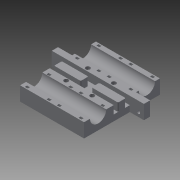
# Autodesk Inventor part: x-carriage
Saved by Autodesk Inventor 2015 SP2 (Build 190223200, 223)
## iProperties
Created: 2016-02-13
Part Number: x-carriage
Material: Generic
Document SubType Name: Modeling
Designer: marc
Density: 1 g/cm^3
Appearance: Default
Author: marc
Autodesk Inventor part; units mm, degrees
ref_plane "YZ Plane" through (0, 0, 0) normal (1, 0, 0) x (0, 1, 0)
ref_plane "XZ Plane" through (0, 0, 0) normal (0, 1, 0) x (-1, 0, 0)
ref_plane "XY Plane" through (0, 0, 0) normal (0, 0, 1) x (1, 0, 0)
sketch "Sketch1" plane through (0, 0, 0) normal (0, 0, 1) x (1, 0, 0)
  line L0 (-42.5, -35) -> (42.5, -35)
  line L1 (42.5, -35) -> (42.5, 35)
  line L2 (42.5, 35) -> (-42.5, 35)
  line L3 (-42.5, 35) -> (-42.5, -35)
  line L4 (-42.5, -35) -> (42.5, 35) construction
  line L5 (42.5, -35) -> (-42.5, 35) construction
  point P0 (0, 0)
  dimension "d0" = 85
  dimension "d1" = 70
  constraints: 12 end point, 2 midpoint, 2 parallel, 1 horizontal, 1 perpendicular
  measures "d0" distance of L1.end L2.end
  measures "d1" distance between parallel lines of L0 L2
extrude "Extrusion1" add sketch "Sketch1" along normal blind 13
sketch "Sketch2" plane through (0, 0, 13) normal (0, 0, 1) x (1, 0, 0)
  line L0 (-42.5, 35) -> (-29.5, 35)
  line L1 (-29.5, 35) -> (-29.5, 13)
  line L2 (-29.5, 13) -> (-42.5, 13)
  line L3 (-42.5, 13) -> (-42.5, 35)
  line L4 (-42.5, -35) -> (-29.5, -35)
  line L5 (-29.5, -35) -> (-29.5, 7.25)
  line L6 (-29.5, 7.25) -> (-42.5, 7.25)
  line L7 (-42.5, 7.25) -> (-42.5, -35)
  line L8 (42.5, 35) -> (-42.5, 35) construction
  line L9 (0, 35) -> (0, -35) construction
  line L10 (-42.5, -35) -> (42.5, -35) construction
  line L11 (42.5, 35) -> (29.5, 35)
  line L12 (29.5, 35) -> (29.5, 13)
  line L13 (29.5, 13) -> (42.5, 13)
  line L14 (42.5, 13) -> (42.5, 35)
  line L15 (42.5, -35) -> (29.5, -35)
  line L16 (29.5, -35) -> (29.5, 7.25)
  line L17 (29.5, 7.25) -> (42.5, 7.25)
  line L18 (42.5, 7.25) -> (42.5, -35)
  point P0 (0, 0)
  dimension "d4" = 13
  dimension "d5" = 5.75
  dimension "d6" = 22
  constraints: 34 end point, 6 symmetric about line, 4 parallel, 2 horizontal, 2 midpoint, 2 perpendicular, 2 point on line
  measures "d4" distance of L1.end L2.end
  measures "d5" distance between parallel lines of L6 L2
  measures "d6" distance of L0.end L1.end
extrude "Extrusion2" cut sketch "Sketch2" against normal through all
sketch "Sketch3" plane through (29.5, 13, 13) normal (1, 0, 0) x (0, 0, -1)
  circle A0 centre (0, 10) radius 7.5
  circle A1 centre (0, -35) radius 7.5
  line L0 (0, 10) -> (0, -35) construction
  line L1 (0, -48) -> (0, -5.75) construction
  line L2 (0, 0) -> (0, 22) construction
  line L3 (0, 22) -> (13, 22) construction
  point P0 (13, -13)
  dimension "d9" = 15
  dimension "d10" = 15
  dimension "d11" = 45
  dimension "d12" = 12
  constraints: 2 centre point, 2 end point, 1 collinear, 1 point on line, 1 vertical
  measures "d9" diameter of A0
  measures "d10" diameter of A1
  measures "d11" distance of L0.end L0.start
  measures "d12" distance from line of L0.start L3
extrude "Extrusion3" cut sketch "Sketch3" against normal through all
sketch "Sketch4" plane through (0, 0, 13) normal (0, 0, 1) x (1, 0, 0)
  line L0 (-12, -10) -> (12, -10) construction
  line L1 (12, -10) -> (12, 10) construction
  line L2 (12, 10) -> (-12, 10) construction
  line L3 (-12, 10) -> (-12, -10) construction
  line L4 (-12, -10) -> (12, 10) construction
  line L5 (12, -10) -> (-12, 10) construction
  point P0 (0, 0)
  dimension "d15" = 24
  dimension "d16" = 20
  constraints: 12 end point, 4 coincident, 2 midpoint, 2 parallel, 1 horizontal, 1 perpendicular
  measures "d15" distance between parallel lines of L1 L3
  measures "d16" distance between parallel lines of L0 L2
hole "Hole1" at (-12, 10, 13) at (12, 10, 13) at (12, -10, 13) at (-12, -10, 13) direction (0, 0, -1) diameter 4 end through all
sketch "Sketch6" plane through (0, 0, 13) normal (0, 0, 1) x (1, 0, 0)
  line L0 (0, -28.0217) -> (0, 47.4955) construction
  line L1 (-24.75, 13) -> (-4.75, 13) construction
  line L2 (-4.75, 13) -> (-4.75, 33) construction
  line L3 (-4.75, 33) -> (-24.75, 33) construction
  line L4 (-24.75, 33) -> (-24.75, 13) construction
  line L5 (-24.75, 13) -> (-4.75, 33) construction
  line L6 (-4.75, 13) -> (-24.75, 33) construction
  line L7 (-26.1, 32) -> (-23.4, 32)
  line L8 (-23.4, 32) -> (-23.4, 34)
  line L9 (-23.4, 34) -> (-26.1, 34)
  line L10 (-26.1, 34) -> (-26.1, 32)
  line L11 (-26.1, 32) -> (-23.4, 34) construction
  line L12 (-23.4, 32) -> (-26.1, 34) construction
  line L13 (-6.1, 32) -> (-3.4, 32)
  line L14 (-3.4, 32) -> (-3.4, 34)
  line L15 (-3.4, 34) -> (-6.1, 34)
  line L16 (-6.1, 34) -> (-6.1, 32)
  line L17 (-6.1, 32) -> (-3.4, 34) construction
  line L18 (-3.4, 32) -> (-6.1, 34) construction
  line L19 (-26.1, 12) -> (-23.4, 12)
  line L20 (-23.4, 12) -> (-23.4, 14)
  line L21 (-23.4, 14) -> (-26.1, 14)
  line L22 (-26.1, 14) -> (-26.1, 12)
  line L23 (-26.1, 12) -> (-23.4, 14) construction
  line L24 (-23.4, 12) -> (-26.1, 14) construction
  line L25 (-6.1, 12) -> (-3.4, 12)
  line L26 (-3.4, 12) -> (-3.4, 14)
  line L27 (-3.4, 14) -> (-6.1, 14)
  line L28 (-6.1, 14) -> (-6.1, 12)
  line L29 (-6.1, 12) -> (-3.4, 14) construction
  line L30 (-3.4, 12) -> (-6.1, 14) construction
  line L31 (-24.75, -33) -> (-4.75, -33) construction
  line L32 (-4.75, -33) -> (-4.75, -13) construction
  line L33 (-4.75, -13) -> (-24.75, -13) construction
  line L34 (-24.75, -13) -> (-24.75, -33) construction
  line L35 (-24.75, -33) -> (-4.75, -13) construction
  line L36 (-4.75, -33) -> (-24.75, -13) construction
  line L37 (-6.1, -14) -> (-3.4, -14)
  line L38 (-3.4, -14) -> (-3.4, -12)
  line L39 (-3.4, -12) -> (-6.1, -12)
  line L40 (-6.1, -12) -> (-6.1, -14)
  line L41 (-6.1, -14) -> (-3.4, -12) construction
  line L42 (-3.4, -14) -> (-6.1, -12) construction
  line L43 (-26.1, -14) -> (-23.4, -14)
  line L44 (-23.4, -14) -> (-23.4, -12)
  line L45 (-23.4, -12) -> (-26.1, -12)
  line L46 (-26.1, -12) -> (-26.1, -14)
  line L47 (-26.1, -14) -> (-23.4, -12) construction
  line L48 (-23.4, -14) -> (-26.1, -12) construction
  line L49 (-26.1, -34) -> (-23.4, -34)
  line L50 (-23.4, -34) -> (-23.4, -32)
  line L51 (-23.4, -32) -> (-26.1, -32)
  line L52 (-26.1, -32) -> (-26.1, -34)
  line L53 (-26.1, -34) -> (-23.4, -32) construction
  line L54 (-23.4, -34) -> (-26.1, -32) construction
  line L55 (-6.1, -34) -> (-3.4, -34)
  line L56 (-3.4, -34) -> (-3.4, -32)
  line L57 (-3.4, -32) -> (-6.1, -32)
  line L58 (-6.1, -32) -> (-6.1, -34)
  line L59 (-6.1, -34) -> (-3.4, -32) construction
  line L60 (-3.4, -34) -> (-6.1, -32) construction
  line L61 (26.1, 32) -> (23.4, 32)
  line L62 (23.4, 32) -> (23.4, 34)
  line L63 (23.4, 34) -> (26.1, 34)
  line L64 (26.1, 34) -> (26.1, 32)
  line L65 (6.1, 32) -> (3.4, 32)
  line L66 (3.4, 32) -> (3.4, 34)
  line L67 (3.4, 34) -> (6.1, 34)
  line L68 (6.1, 34) -> (6.1, 32)
  line L69 (26.1, 12) -> (23.4, 12)
  line L70 (23.4, 12) -> (23.4, 14)
  line L71 (23.4, 14) -> (26.1, 14)
  line L72 (26.1, 14) -> (26.1, 12)
  line L73 (6.1, 12) -> (3.4, 12)
  line L74 (3.4, 12) -> (3.4, 14)
  line L75 (3.4, 14) -> (6.1, 14)
  line L76 (6.1, 14) -> (6.1, 12)
  line L77 (6.1, -14) -> (3.4, -14)
  line L78 (3.4, -14) -> (3.4, -12)
  line L79 (3.4, -12) -> (6.1, -12)
  line L80 (6.1, -12) -> (6.1, -14)
  line L81 (26.1, -14) -> (23.4, -14)
  line L82 (23.4, -14) -> (23.4, -12)
  line L83 (23.4, -12) -> (26.1, -12)
  line L84 (26.1, -12) -> (26.1, -14)
  line L85 (26.1, -34) -> (23.4, -34)
  line L86 (23.4, -34) -> (23.4, -32)
  line L87 (23.4, -32) -> (26.1, -32)
  line L88 (26.1, -32) -> (26.1, -34)
  line L89 (6.1, -34) -> (3.4, -34)
  line L90 (3.4, -34) -> (3.4, -32)
  line L91 (3.4, -32) -> (6.1, -32)
  line L92 (6.1, -32) -> (6.1, -34)
  point P0 (0, 0)
  point P1 (-14.75, 23)
  point P2 (-14.75, -23)
  dimension "d24" = 14.75
  dimension "d25" = 23
  dimension "d26" = 20
  dimension "d27" = 20
  dimension "d28" = 2.7
  dimension "d29" = 2
  dimension "d30" = 14.75
  dimension "d31" = 20
  dimension "d32" = 20
  dimension "d33" = 23
  dimension "d34" = 2.7
  dimension "d35" = 2
  constraints: 186 end point, 32 symmetric about line, 20 midpoint, 20 parallel, 10 horizontal, 10 perpendicular, 9 equal length, 7 point on line, 1 vertical
  measures "d24" distance from line of L0 point (-14.75, 23)
  measures "d25" vertical distance of point (0, 0) point (-14.75, 23)
  measures "d26" distance of L3.end L1.start
  measures "d27" distance between parallel lines of L2 L4
  measures "d28" distance of L8.end L9.end
  measures "d29" distance between parallel lines of L7 L9
  measures "d30" distance from line of L0 point (-14.75, -23)
  measures "d31" distance of L31.start L31.end
  measures "d32" distance between parallel lines of L31 L33
  measures "d33" vertical distance of point (0, 0) point (-14.75, -23)
  measures "d34" distance of L44.end L45.end
  measures "d35" distance between parallel lines of L43 L45
extrude "Extrusion4" cut sketch "Sketch6" against normal through all
sketch "Sketch7" plane through (0, 0, 13) normal (0, 0, 1) x (1, 0, 0)
  line L0 (-42.3851, 7.25) -> (42.4952, 7.25) construction
  line L1 (-42.5, 7.25) -> (-29.5, 7.25) projected
  line L2 (-42.3851, 0) -> (42.4952, 0) construction
  line L3 (-29.5, 7.25) -> (-29.5, -14.5) projected
  line L4 (-29.5, 3.5) -> (-5, 3.5)
  line L5 (-5, 3.5) -> (-5, -3.625)
  line L6 (-5, -3.625) -> (-29.5, -3.625)
  line L7 (-29.5, -3.625) -> (-29.5, -7.625)
  line L8 (-29.5, -7.625) -> (29.5, -7.625)
  line L9 (29.5, 7.25) -> (29.5, -35) projected
  line L10 (29.5, -7.625) -> (29.5, -3.625)
  line L11 (29.5, -3.625) -> (5, -3.625)
  line L12 (5, -3.625) -> (5, 3.5)
  line L13 (5, 3.5) -> (29.5, 3.5)
  line L14 (29.5, 3.5) -> (29.5, 7.25)
  line L15 (29.5, 7.25) -> (-29.5, 7.25)
  line L16 (-29.5, 7.25) -> (-29.5, 3.5)
  line L17 (0, 0) -> (0, 21.6097) construction
  dimension "d40" = 4
  dimension "d42" = 5
  dimension "d57" = 3.75
  constraints: 30 end point, 10 point on line, 4 collinear, 4 horizontal, 4 perpendicular, 1 midpoint, 1 vertical, 1 other
  measures "d40" distance between parallel lines of L8 L6
  measures "d42" distance from line of L17.start L5
  measures "d57" distance between parallel lines of L4 L0
extrude "Extrusion5" cut sketch "Sketch7" against normal blind 7.5 contours L15 L9 L13 L12 L11 L8 L3 L6 L5 L4
sketch "Sketch8" plane through (-42.5, 13, 13) normal (0, 1, 0) x (1, 0, 0)
  line L0 (42.5, 13) -> (42.5, -23.2157) construction
  line L1 (72, 13) -> (13, 13) construction
  line L2 (0, 0) -> (0, 13) construction
  point P0 (5, 9)
  point P1 (80, 9)
  dimension "d45" = 4
  dimension "d46" = 5
  constraints: 2 end point, 1 symmetric about line, 1 vertical
  measures "d45" distance from line of L1 point (5, 9)
  measures "d46" distance from line of L2 point (5, 9)
hole "Hole2" at (-37.5, 13, 4) at (37.5, 13, 4) direction (0, -1, 0) diameter 3 end through all
sketch "Sketch9" plane through (0, 0, 0) normal (0, 0, -1) x (-1, 0, 0)
  line L0 (-26.1, 32) -> (-23.4, 32)
  line L1 (-23.4, 32) -> (-23.4, 14)
  line L2 (-23.4, 14) -> (-26.1, 14)
  line L3 (-26.1, 14) -> (-26.1, 32)
  line L4 (-6.1, 32) -> (-3.4, 32)
  line L5 (-3.4, 32) -> (-3.4, 14)
  line L6 (-3.4, 14) -> (-6.1, 14)
  line L7 (-6.1, 14) -> (-6.1, 32)
  line L8 (-26.1, -14) -> (-23.4, -14)
  line L9 (-23.4, -14) -> (-23.4, -32)
  line L10 (-23.4, -32) -> (-26.1, -32)
  line L11 (-26.1, -32) -> (-26.1, -14)
  line L12 (-6.1, -14) -> (-3.4, -14)
  line L13 (-3.4, -14) -> (-3.4, -32)
  line L14 (-3.4, -32) -> (-6.1, -32)
  line L15 (-6.1, -32) -> (-6.1, -14)
  line L16 (3.4, 32) -> (6.1, 32)
  line L17 (6.1, 32) -> (6.1, 14)
  line L18 (6.1, 14) -> (3.4, 14)
  line L19 (3.4, 14) -> (3.4, 32)
  line L20 (23.4, 32) -> (26.1, 32)
  line L21 (26.1, 32) -> (26.1, 14)
  line L22 (26.1, 14) -> (23.4, 14)
  line L23 (23.4, 14) -> (23.4, 32)
  line L24 (3.4, -14) -> (6.1, -14)
  line L25 (6.1, -14) -> (6.1, -32)
  line L26 (6.1, -32) -> (3.4, -32)
  line L27 (3.4, -32) -> (3.4, -14)
  line L28 (3.4, -14) -> (3.4, -12) projected
  line L29 (23.4, -14) -> (26.1, -14)
  line L30 (26.1, -14) -> (26.1, -32)
  line L31 (26.1, -32) -> (23.4, -32)
  line L32 (23.4, -32) -> (23.4, -14)
  line L33 (23.4, -14) -> (23.4, -12) projected
  line L34 (26.1, -14) -> (23.4, -14) projected
  line L35 (6.1, -14) -> (3.4, -14) projected
  point P0 (0, 0)
  constraints: 64 end point, 16 parallel, 8 horizontal, 8 perpendicular, 4 collinear, 1 coincident
extrude "Extrusion6" cut sketch "Sketch9" against normal blind 2
fillet "Fillet1" radius 1 8 edges at (-5, -3.625, 9.25) (-5, 3.5, 9.25) (5, 3.5, 9.25) (5, -3.625, 9.25) (29.5, -3.625, 9.25) (29.5, 3.5, 9.25) (-29.5, -3.625, 9.25) (-29.5, 3.5, 9.25)
body "Solid1"
